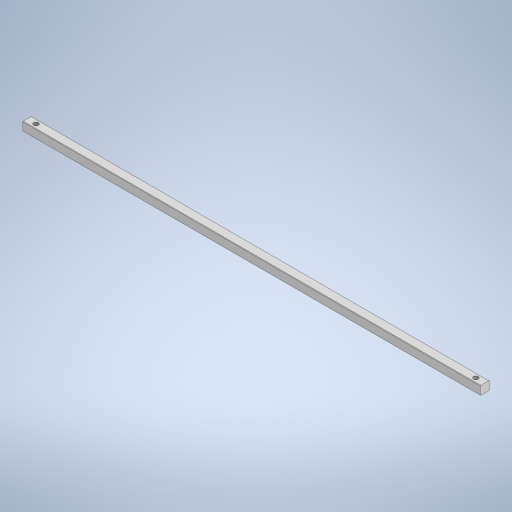
# Autodesk Inventor part: Scraper Cross Brace
Saved by Autodesk Inventor 2024.2 (Build 282272000, 272)
## iProperties
Created: 2025-11-04
Part Number: Scraper Cross Brace
Material: Generic
Document SubType Name: Modeling
Designer: thero
Density: 1 g/cm^3
Appearance: Default
Author: Theron Tyler
Title: Scraper Cross Brace
Autodesk Inventor part; units mm, degrees
ref_plane "YZ Plane" through (0, 0, 0) normal (1, 0, 0) x (0, 1, 0)
ref_plane "XZ Plane" through (0, 0, 0) normal (0, 1, 0) x (-1, 0, 0)
ref_plane "XY Plane" through (0, 0, 0) normal (0, 0, 1) x (1, 0, 0)
sketch "Sketch1" plane through (0, 0, 0) normal (1, 0, 0) x (0, 1, 0)
  line L0 (0, 0) -> (6.35, 0)
  line L1 (6.35, 0) -> (6.35, -6.35)
  line L2 (6.35, -6.35) -> (0, -6.35)
  line L3 (0, -6.35) -> (0, 0)
  dimension "d0" = 6.35
  dimension "d1" = 6.35
  constraints: 8 end point, 2 parallel, 1 horizontal, 1 perpendicular
  measures "d0" distance of L1.end L2.end
  measures "d1" distance of L0.end L1.end
extrude "Extrusion1" add sketch "Sketch1" along normal blind 330.2
fillet "Fillet1" radius 0.3175 4 edges at (165.1, 6.35, 0) (165.1, 6.35, -6.35) (165.1, 0, -6.35) (165.1, 0, 0)
sketch "Sketch2" plane through (0, 6.35, -6.0325) normal (0, 1, 0) x (1, 0, 0)
  circle A0 centre (6.35, -2.8575) radius 1.7859
  line L0 (0, 0) -> (0, -5.715) projected
  circle A1 centre (323.85, -2.8575) radius 1.7859
  line L1 (330.2, 0) -> (330.2, -5.715) projected
  point P0 (0, -6.0325)
  dimension "d5" = 3.5719
  dimension "d6" = 6.35
  dimension "d7" = 3.5719
  dimension "d8" = 6.35
  constraints: 2 centre point
  measures "d5" diameter of A0
  measures "d6" distance from line of L0 A0.centre
  measures "d7" diameter of A1
  measures "d8" distance from line of L1 A1.centre
extrude "Extrusion2" cut sketch "Sketch2" against normal blind 6.35
thread "Thread1" size "8-32 UNC" class "2B" standard "ANSI Unified Screw Threads" full length
thread "Thread2" size "8-32 UNC" class "2B" standard "ANSI Unified Screw Threads" full length
body "Solid1"
